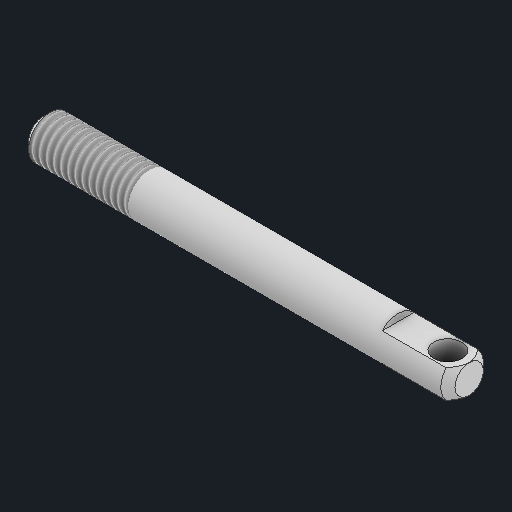
# Autodesk Inventor part: M6x1_THREADED_ROD_CPY
Saved by Autodesk Inventor 2023 (Build 270158000, 158)
## iProperties
Created: 2023-02-24
Part Number: M6x1_THREADED_ROD_CPY
Material: Generic
Document SubType Name: Modeling
Designer: roota
Density: 1 g/cm^3
Appearance: Default
Author: roota
Autodesk Inventor part; units mm, degrees
ref_plane "YZ Plane" through (0, 0, 0) normal (1, 0, 0) x (0, 1, 0)
ref_plane "XZ Plane" through (0, 0, 0) normal (0, 1, 0) x (-1, 0, 0)
ref_plane "XY Plane" through (0, 0, 0) normal (0, 0, 1) x (1, 0, 0)
sketch "Sketch1" plane through (0, 0, 0) normal (0, 0, 1) x (1, 0, 0)
  line L0 (0, 0) -> (60, 0)
  line L1 (60, 0) -> (60, 3)
  line L2 (60, 3) -> (0, 3)
  line L3 (0, 3) -> (0, 0)
  dimension "d0" = 60
  dimension "d1" = 6
  constraints: 8 end point, 2 parallel, 1 horizontal, 1 perpendicular
  measures "d0" distance of L2.end L1.end
  measures "d1" diameter of L2 L0
revolve "Revolution1" add sketch "Sketch1" angle 360 about axis through (0, 0, 0) along (1, 0, 0)
thread "Thread1" size "M6x1" class "6g" standard "ANSI Metric M Profile" length 15
chamfer "Chamfer1" distance 1 angle 45 2 edges at (0, -3, 0) (60, -3, 0)
sketch "Sketch2" plane through (0, 0, 0) normal (0, 0, 1) x (1, 0, 0)
  line L0 (1, 3) -> (59, 3) projected
  line L1 (60, 3) -> (50, 3)
  line L2 (50, 3) -> (50, 2)
  line L3 (50, 2) -> (60, 2)
  line L4 (60, 2) -> (60, 3)
  line L5 (60, -3) -> (60, 3) projected
  line L6 (60, -3) -> (50, -3)
  line L7 (50, -3) -> (50, -2)
  line L8 (50, -2) -> (60, -2)
  line L9 (60, -2) -> (60, -3)
  point P0 (0, 0)
  point P1 (50, 3)
  dimension "d8" = 4
  dimension "d15" = 10
  constraints: 16 end point, 4 parallel, 2 equal length, 2 horizontal, 2 perpendicular, 2 point on line, 1 other
  measures "d8" distance between parallel lines of L3 L8
  measures "d15" distance of L6.start L6.end
extrude "Extrusion1" cut sketch "Sketch2" along normal through all both and the other way through all
sketch "Sketch3" plane through (50, -2, -2.2361) normal (0, -1, 0) x (1, 0, 0)
  circle A0 centre (7, 2.2361) radius 2
  line L0 (10, 2.2361) -> (10, 0.2361) projected
  point P0 (-50, 2.2361)
  dimension "d11" = 4
  dimension "d14" = 3
  constraints: 1 centre point
  measures "d11" diameter of A0
  measures "d14" distance from line of L0 A0.centre
extrude "Extrusion2" cut sketch "Sketch3" against normal through all
body "Solid1"
